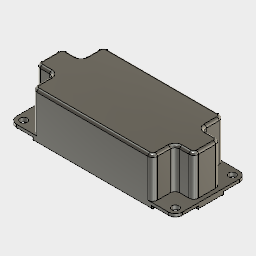
3351 Enclosed Speaker 3W 4Ohm (Autodesk Fusion 360 design; units mm, degrees)
Autodesk Fusion 360 part; units mm, degrees
sketch "Sketch1" plane through (0, 0, 0) normal (0, 0, 1) x (1, 0, 0)
  line L0 (0, 0) -> (70, 0)
  line L1 (70, 0) -> (70, 30)
  line L2 (70, 30) -> (0, 30)
  line L3 (0, 30) -> (0, 0)
  line L4 (35, 30) -> (35, 0) construction
  line L5 (0, 15) -> (70, 15) construction
  line L6 (67, 3) -> (3, 3) construction
  line L7 (3, 3) -> (3, 27) construction
  line L8 (3, 27) -> (67, 27) construction
  line L9 (67, 27) -> (67, 3) construction
  line L10 (67, 3) -> (3, 27) construction
  line L11 (3, 3) -> (67, 27) construction
  circle A0 centre (3, 27) radius 1.5
  circle A1 centre (67, 27) radius 1.5
  circle A2 centre (3, 3) radius 1.5
  circle A3 centre (67, 3) radius 1.5
  line L12 (0, 30) -> (9.6, 30)
  line L13 (9.6, 30) -> (9.6, 20.6)
  line L14 (9.6, 20.6) -> (0, 20.6)
  line L15 (0, 20.6) -> (0, 30)
  line L16 (60.4, 20.6) -> (70, 20.6)
  line L17 (60.4, 30) -> (60.4, 20.6)
  line L18 (9.6, 0) -> (9.6, 9.4)
  line L19 (9.6, 9.4) -> (0, 9.4)
  line L20 (60.4, 0) -> (60.4, 9.4)
  line L21 (60.4, 9.4) -> (70, 9.4)
  line L22 (1.7, 20.6) -> (1.7, 9.4)
  line L23 (68.3, 20.6) -> (68.3, 9.4)
  point P0 (35, 15)
  dimension "d1" = 70
  dimension "d2" = 30
  dimension "d6" = 64
  dimension "d7" = 24
  dimension "d8" = 3
  dimension "d9" = 9.6
  dimension "d10" = 9.4
  dimension "d14" = 1.7
  measures "d1" distance of L0.start L0.end
  measures "d2" distance of L0.start L2.end
  measures "d6" distance of L7.end L8.end
  measures "d7" distance of L6.end L7.end
  measures "d8" diameter of A0
  measures "d9" distance of L2.end L12.end
  measures "d10" distance of L2.end L14.end
  measures "d14" distance of L3 L22
extrude "Extrude1" add sketch "Sketch1" along normal blind 2.7
fillet "Fillet1" radius 3 4 edges at (70, 0, 1.35) (0, 30, 1.35) (70, 30, 1.35) (0, 0, 1.35)
extrude "Extrude2" add sketch "Sketch1" along normal blind 19.7 contours L0 L2 L13 L14 L16 L17 L18 L19 L20 L21 L22 L23
fillet "Fillet2" radius 2 12 edges at (60.4, 30, 11.2) (68.3, 9.4, 11.2) (60.4, 9.4, 11.2) (1.7, 20.6, 11.2) (9.6, 20.6, 11.2) (9.6, 30, 11.2) (68.3, 20.6, 11.2) (60.4, 0, 11.2) (60.4, 20.6, 11.2) (1.7, 9.4, 11.2) (9.6, 0, 11.2) (9.6, 9.4, 11.2)
fillet "Fillet3" radius 1 24 edges at (5.65, 20.6, 19.7) (9.0142, 21.1858, 19.7) (9.6, 25.3, 19.7) (10.1858, 29.4142, 19.7) (35, 30, 19.7) (59.8142, 29.4142, 19.7) (60.4, 25.3, 19.7) (60.9858, 21.1858, 19.7) (64.35, 20.6, 19.7) (67.7142, 20.0142, 19.7) (68.3, 15, 19.7) (67.7142, 9.9858, 19.7) (64.35, 9.4, 19.7) (60.9858, 8.8142, 19.7) (60.4, 4.7, 19.7) (59.8142, 0.5858, 19.7) (35, 0, 19.7) (10.1858, 0.5858, 19.7) (9.6, 4.7, 19.7) (9.0142, 8.8142, 19.7) (5.65, 9.4, 19.7) (2.2858, 9.9858, 19.7) (1.7, 15, 19.7) (2.2858, 20.0142, 19.7)
extrude "Extrude3" cut sketch "Sketch1" along normal blind 1 contours L0 L3 L18 L19 | L0 L1 L20 L21 | L2 L3 L12 L13 L14 L15 | L1 L2 L16 L17
fillet "Fillet4" radius 2 4 edges at (9.6, 20.6, 0.5) (9.6, 9.4, 0.5) (60.4, 9.4, 0.5) (60.4, 20.6, 0.5)
fillet "Fillet5" radius 0.5 36 edges at (66.2, 9.4, 0) (60.9858, 8.8142, 0) (60.4, 3.7, 0) (60.4, 26.3, 0) (60.9858, 21.1858, 0) (66.2, 20.6, 0) (9.6, 3.7, 0) (9.0142, 8.8142, 0) (3.8, 9.4, 0) (3.8, 20.6, 0) (9.0142, 21.1858, 0) (9.6, 26.3, 0) (35, 0, 0) (35, 30, 0) (6.3, 30, 1) (0.8787, 29.1213, 1) (0, 23.8, 1) (0, 6.2, 1) (0.8787, 0.8787, 1) (6.3, 0, 1) (63.7, 0, 1) (69.1213, 0.8787, 1) (70, 6.2, 1) (70, 23.8, 1) (69.1213, 29.1213, 1) (63.7, 30, 1) (70, 15, 0) (0, 15, 0) (70, 9.4, 0.5) (70, 20.6, 0.5) (0, 20.6, 0.5) (60.4, 30, 0.5) (0, 9.4, 0.5) (9.6, 0, 0.5) (9.6, 30, 0.5) (60.4, 0, 0.5)
sketch "Sketch2" plane through (0, 0, 0) normal (0, 0, -1) x (1, 0, 0)
  line L0 (59.9, -0.5) -> (10.1, -0.5)
  line L1 (10.1, -0.5) -> (10.1, -7.4)
  arc A0 (7.6, -9.9) -> (10.1, -7.4) centre (7.6, -7.4) ccw
  line L2 (7.6, -9.9) -> (0.5, -9.9)
  line L3 (0.5, -9.9) -> (0.5, -20.1)
  line L4 (0.5, -20.1) -> (7.6, -20.1)
  arc A1 (10.1, -22.6) -> (7.6, -20.1) centre (7.6, -22.6) ccw
  line L5 (10.1, -22.6) -> (10.1, -29.5)
  line L6 (10.1, -29.5) -> (59.9, -29.5)
  line L7 (59.9, -29.5) -> (59.9, -22.6)
  arc A2 (62.4, -20.1) -> (59.9, -22.6) centre (62.4, -22.6) ccw
  line L8 (62.4, -20.1) -> (69.5, -20.1)
  line L9 (69.5, -20.1) -> (69.5, -9.9)
  line L10 (69.5, -9.9) -> (62.4, -9.9)
  arc A3 (59.9, -7.4) -> (62.4, -9.9) centre (62.4, -7.4) ccw
  line L11 (59.9, -7.4) -> (59.9, -0.5)
  line L12 (69.5, -15) -> (0.5, -15) construction
  line L13 (12.35, -1.5) -> (50.65, -1.5)
  line L14 (50.65, -1.5) -> (50.65, -28.5)
  line L15 (50.65, -28.5) -> (12.35, -28.5)
  line L16 (12.35, -28.5) -> (12.35, -1.5)
  line L17 (12.35, -1.5) -> (50.65, -28.5) construction
  line L18 (50.65, -1.5) -> (12.35, -28.5) construction
  line L19 (0, -9.9) -> (0, -20.1)
  point P0 (31.5, -15)
  dimension "d24" = 38.3
  dimension "d25" = 27
  dimension "d26" = 31.5
  measures "d24" distance of L14.end L15.end
  measures "d25" distance of L13.end L14.end
  measures "d26" distance of P0 L19
extrude "Extrude4" cut sketch "Sketch2" against normal blind 2 contours L13 L14 L15 L16
fillet "Fillet6" radius 13.5 4 edges at (12.35, 1.5, 1) (12.35, 28.5, 1) (50.65, 1.5, 1) (50.65, 28.5, 1)
sketch "Sketch3" plane through (0, 0, 2) normal (0, 0, -1) x (1, 0, 0)
  arc A0 (37.15, -28.5) -> (37.15, -1.5) centre (37.15, -15) ccw
  line L0 (37.15, -1.5) -> (25.85, -1.5)
  arc A1 (25.85, -1.5) -> (25.85, -28.5) centre (25.85, -15) ccw
  line L1 (25.85, -28.5) -> (37.15, -28.5)
  line L2 (31.5, -1.5) -> (31.5, -28.5) construction
  line L3 (12.35, -15) -> (50.65, -15) construction
  circle A2 centre (31.5, -15) radius 7.45
  arc A3 (37.15, -26.5) -> (37.15, -3.5) centre (37.15, -15) ccw
  line L4 (37.15, -3.5) -> (25.85, -3.5)
  arc A4 (25.85, -3.5) -> (25.85, -26.5) centre (25.85, -15) ccw
  line L5 (25.85, -26.5) -> (37.15, -26.5)
  line L6 (25.85, -25) -> (37.15, -25)
  arc A5 (37.15, -25) -> (37.15, -5) centre (37.15, -15) ccw
  line L7 (37.15, -5) -> (25.85, -5)
  arc A6 (25.85, -5) -> (25.85, -25) centre (25.85, -15) ccw
  circle A7 centre (31.5, -15) radius 5.95
  dimension "d30" = 14.9
  dimension "d31" = 1.5
  dimension "d35" = 2
  dimension "d36" = 3.5
  measures "d30" diameter of A2
extrude "Extrude5" add sketch "Sketch3" along normal blind 1 contours A2
fillet "Fillet7" radius 0.75 2 edges at (25.9527, 12.8484, 1) (24.5542, 17.694, 1)
extrude "Extrude6" cut sketch "Sketch3" against normal blind 1 contours A3 L4 A4 L5
fillet "Fillet8" radius 1 8 edges at (48.65, 15, 2) (31.5, 26.5, 2) (14.35, 15, 2) (31.5, 3.5, 2) (47.15, 15, 2) (31.5, 5, 2) (15.85, 15, 2) (31.5, 25, 2)
equation "d11 = 2.7 mm + 17 mm"
